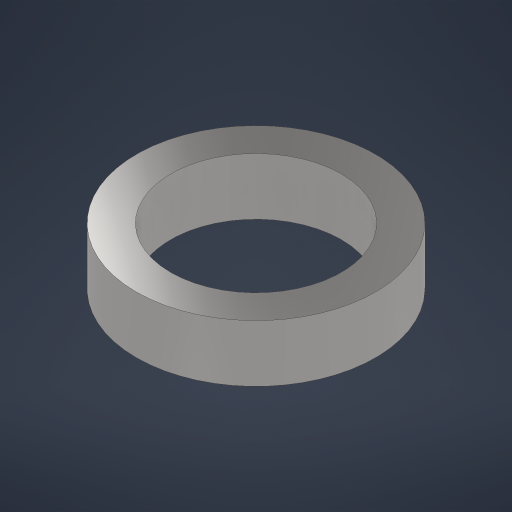
# Autodesk Inventor part: Bearing_GB
Saved by Autodesk Inventor 2024.2 (Build 282272000, 272)
## iProperties
Created: 2026-01-03
Part Number: Bearing_GB
Material: Stainless Steel
Document SubType Name: Modeling
Designer: 4aida
Density: 8 g/cm^3
Appearance: Semi-Polished
Author: 4aida
Autodesk Inventor part; units mm, degrees
ref_plane "YZ Plane" through (0, 0, 0) normal (1, 0, 0) x (0, 1, 0)
ref_plane "XZ Plane" through (0, 0, 0) normal (0, 1, 0) x (-1, 0, 0)
ref_plane "XY Plane" through (0, 0, 0) normal (0, 0, 1) x (1, 0, 0)
sketch "Sketch2" plane through (0, 0, 0) normal (1, 0, 0) x (0, 1, 0)
  line L0 (2.5, 10.5) -> (-2.5, 10.5)
  line L1 (-2.5, 10.5) -> (-2.5, 7.5)
  line L2 (-2.5, 7.5) -> (2.5, 7.5)
  line L3 (2.5, 7.5) -> (2.5, 10.5)
  line L4 (2.5, 0) -> (-2.5, 0)
  point P0 (0, 0)
  point P1 (0, 0)
  dimension "d0" = 5
  dimension "d1" = 15
  dimension "d2" = 21
  constraints: 10 end point, 2 horizontal, 2 parallel, 2 vertical alignment, 1 coincident, 1 midpoint, 1 perpendicular
  measures "d0" distance of L0.start L0.end
  measures "d1" diameter of L2 L4
  measures "d2" diameter of L0 L4
revolve "Revolution1" add sketch "Sketch2" angle 360 about axis through (0, 2.5, 0) along (0, -1, 0)
body "Solid1"
